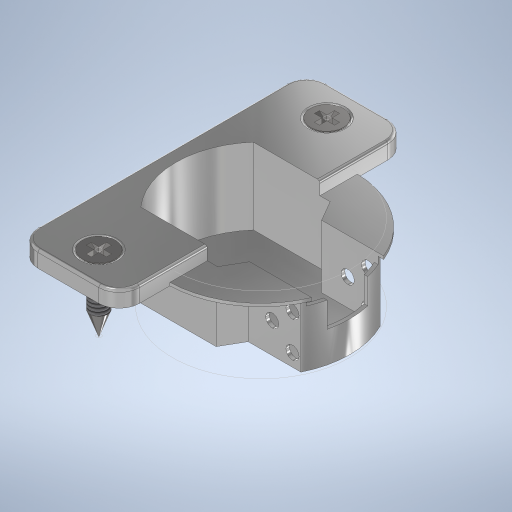
# Autodesk Inventor part: Cup for hinge with wood screws
Saved by Autodesk Inventor 2024 (Build 280153000, 153)
## iProperties
Created: 2007-06-13
Document SubType Name: Modeling
Designer: G.K.
Authority: Design by UAB Čeli APS
Material: Steel
Mass: 17.6743 g
Surface Area: 66.7103 cm^2
Volume: 2.2515 cm^3
Density: 7.85 g/cm^3
Appearance: Chrome - Polished
Part Number: Cup for hinge with wood screws
Perskaiciuoti: 1
Mase: 0.01767427
Autodesk Inventor part; units mm, degrees
ref_plane "YZ Plane" through (0, 0, 0) normal (1, 0, 0) x (0, 1, 0)
sketch "Sketch1" plane through (0, 0, 0) normal (0, 0, 1) x (1, 0, 0)
  line L0 (-10, -28.5) -> (10, -28.5)
  line L1 (10, -28.5) -> (10, 28.5)
  line L2 (10, 28.5) -> (-10, 28.5)
  line L3 (-10, 28.5) -> (-10, -28.5)
  point P0 (0, 0)
  point P1 (-10, 0)
  point P2 (0, 28.5)
  dimension "d0" = 20
  dimension "d1" = 57
  constraints: 8 end point, 2 midpoint, 2 parallel, 1 horizontal, 1 horizontal alignment, 1 perpendicular, 1 vertical alignment
  measures "d0" distance between parallel lines of L1 L3
  measures "d1" distance of L2.end L0.start
extrude "Extrusion1" add sketch "Sketch1" along normal blind 3.2
sketch "Sketch2" plane through (0, 0, 3.2) normal (0, 0, 1) x (1, 0, 0)
  line L0 (-10, -28.5) -> (-10, 28.5) projected
  line L1 (10, 28.5) -> (10, -28.5) projected
  line L2 (-10, 28.5) -> (10, 28.5) projected
  line L3 (0, 22.5) -> (0, -22.5) construction
  line L4 (-10, 0) -> (10, 0) construction
  point P0 (0, 0)
  dimension "d4" = 45
  constraints: 4 end point, 3 midpoint, 1 perpendicular, 1 symmetric about line
  measures "d4" distance of L3.start L3.end
hole "Hole1" at (0, -22.5, 3.2) at (0, 22.5, 3.2) direction (0, 0, -1) diameter 4.3 end through all countersink diameter 7 countersink angle 90
fillet "Fillet1" radius 0.5 4 edges at (0, 26, 3.2) (0, -19, 3.2) (0, -20.35, 1.85) (0, 24.65, 1.85)
fillet "Fillet1" radius 4 4 edges at (10, -28.5, 1.6) (-10, -28.5, 1.6) (-10, 28.5, 1.6) (10, 28.5, 1.6)
fillet "Fillet2" radius 0.5 8 edges at (-10, 0, 3.2) (-8.8284, 27.3284, 3.2) (0, 28.5, 3.2) (8.8284, 27.3284, 3.2) (10, 0, 3.2) (8.8284, -27.3284, 3.2) (0, -28.5, 3.2) (-8.8284, -27.3284, 3.2)
shell "Shell1" thickness 0.7 removed faces 1 at (6.9997, 6.8654, 0)
sketch "Sketch3" plane through (0, 0, 0) normal (0, 0, -1) x (-1, 0, 0)
  line L0 (-10, -24.5) -> (-10, 24.5) projected
  arc A0 (-10, 18.4932) -> (-10, -18.4932) centre (-9.5, 0) ccw
  line L1 (-39.6485, 0) -> (14.7113, 0)
  point P0 (0, 0)
  dimension "d16" = 18.5
  dimension "d17" = 0.5
  constraints: 3 point on line, 2 end point, 2 point on circle, 1 centre point, 1 horizontal, 2 other
  measures "d16" radius of A0
  measures "d17" distance from line of L0 A0.centre
extrude "Extrusion2" add sketch "Sketch3" against normal blind 0.6
sketch "Sketch4" plane through (0, 0, 0) normal (0, 0, -1) x (-1, 0, 0)
  line L0 (-14.7486, 7.8) -> (-25.1656, 7.8)
  arc A0 (-25.1656, 7.8) -> (-27, 0) centre (-9.5, 0) ccw
  arc A1 (-27, 0) -> (-25.1656, -7.8) centre (-9.5, 0) ccw
  line L1 (-25.1656, -7.8) -> (-14.7486, -7.8)
  line L2 (-12.4392, 11.8) -> (-14.7486, 7.8)
  line L3 (3.4232, 11.8) -> (-12.4392, 11.8)
  line L4 (-14.7486, -7.8) -> (-12.4392, -11.8)
  line L5 (-12.4392, -11.8) -> (3.4232, -11.8)
  arc A2 (3.4232, -11.8) -> (3.4232, 11.8) centre (-9.5, 0) ccw
  point P0 (0, 0)
  constraints: 12 end point, 6 point on circle, 4 horizontal, 3 centre point, 17 other
extrude "Extrusion3" add sketch "Sketch4" along normal blind 12.5
sketch "Sketch5" plane through (0, 0, 0) normal (0, 0, 1) x (1, 0, 0)
  line L0 (9.3, -11.8) -> (9.3, 11.8) projected
  line L1 (-3.4232, 11.8) -> (9.3, 11.8) projected
  arc A0 (-3.4232, 11.8) -> (-3.4232, -11.8) centre (9.5, 0) ccw projected
  line L2 (9.3, -11.8) -> (-3.4232, -11.8) projected
  point P0 (0, 0)
extrude "Extrusion4" add sketch "Sketch5" along normal up to surface (2.5 mm away)
sketch "Sketch6" plane through (0, 0, 3.2) normal (0, 0, 1) x (1, 0, 0)
  arc A0 (-3.4232, 11.8) -> (-3.4232, -11.8) centre (9.5, 0) ccw projected
  line L0 (9.3, 11.8) -> (-3.4232, 11.8) projected
  line L1 (12.4392, 11.8) -> (9.3, 11.8) projected
  line L2 (14.7486, 7.8) -> (12.4392, 11.8) projected
  line L3 (25.1656, 7.8) -> (14.7486, 7.8) projected
  line L4 (-3.4232, -11.8) -> (9.3, -11.8) projected
  line L5 (9.3, -11.8) -> (12.4392, -11.8) projected
  line L6 (12.4392, -11.8) -> (14.7486, -7.8) projected
  line L7 (14.7486, -7.8) -> (25.1656, -7.8) projected
  arc A1 (25.1656, -7.8) -> (25.1656, 7.8) centre (9.5, 0) ccw projected
  arc A2 (-3.1107, 11.1) -> (-3.1107, -11.1) centre (9.5, 0) ccw
  line L8 (-3.1107, -11.1) -> (9.3, -11.1)
  line L9 (9.3, -11.1) -> (12.035, -11.1)
  line L10 (12.035, -11.1) -> (14.3444, -7.1)
  line L11 (14.3444, -7.1) -> (24.726, -7.1)
  arc A3 (24.726, -7.1) -> (24.726, 7.1) centre (9.5, 0) ccw
  line L12 (24.726, 7.1) -> (14.3444, 7.1)
  line L13 (14.3444, 7.1) -> (12.035, 11.1)
  line L14 (12.035, 11.1) -> (9.3, 11.1)
  line L15 (9.3, 11.1) -> (-3.1107, 11.1)
  dimension "d24" = 0.7
  constraints: 16 end point, 4 point on circle, 2 centre point, 9 other
  measures "d24" radial gap between concentric circles of A2 A0
extrude "Extrusion5" cut sketch "Sketch6" against normal blind 15 contours L15 L14 L13 L12 A3 L11 L10 L9 L8 A2
sketch "Sketch7" plane through (0, 0, 0.6) normal (0, 0, 1) x (1, 0, 0)
  arc A0 (10, -18.4932) -> (10, 18.4932) centre (9.5, 0) ccw projected
  line L0 (14.3444, 7.1) -> (24.726, 7.1) projected
  line L1 (24.726, -7.1) -> (14.3444, -7.1) projected
  line L2 (24, 7.1) -> (28, 7.1)
  line L3 (28, 7.1) -> (28, -7.1)
  line L4 (28, -7.1) -> (24, -7.1)
  line L5 (24, -7.1) -> (24, 7.1)
  point P0 (0, 0)
  dimension "d27" = 4
  constraints: 8 end point, 2 parallel, 1 collinear, 1 horizontal, 1 perpendicular, 1 point on line, 1 tangent
  measures "d27" distance between parallel lines of L5 L3
extrude "Extrusion6" cut sketch "Sketch7" against normal blind 2
sketch "Sketch8" plane through (0, 0, -1.4) normal (0, 0, 1) x (1, 0, 0)
  arc A0 (25.495, -7.1) -> (25.495, 7.1) centre (9.5, 0) ccw projected
  line L0 (-17.4, 0) -> (34.4, 0) projected
  line L1 (23, 4) -> (27, 4)
  line L2 (27, 4) -> (27, -4)
  line L3 (27, -4) -> (23, -4)
  line L4 (23, -4) -> (23, 4)
  point P0 (0, 0)
  dimension "d30" = 8
  dimension "d31" = 4
  constraints: 8 end point, 2 parallel, 1 horizontal, 1 perpendicular, 1 tangent, 1 other
  measures "d30" distance between parallel lines of L3 L1
  measures "d31" distance between parallel lines of L2 L4
extrude "Extrusion7" cut sketch "Sketch8" against normal blind 5
sketch "Sketch9" plane through (14.7486, 7.8, -12.5) normal (0, 1, 0) x (1, 0, 0)
  line L0 (10.417, 0) -> (0, 0) projected
  line L1 (10.417, -12.5) -> (10.417, 0) projected
  line L2 (8.7514, -9.5) -> (8.7514, -2.5) construction
  line L3 (8.7514, -9.5) -> (4.7514, -6) construction
  line L4 (4.7514, -6) -> (8.7514, -2.5) construction
  line L5 (4.7514, -6) -> (8.7514, -6) construction
  line L6 (-24.7486, -12.5) -> (-24.7486, -15.2) projected
  point P0 (-14.7486, -12.5)
  dimension "d35" = 7
  dimension "d36" = 4
  dimension "d37" = 6
  dimension "d38" = 29.5
  constraints: 8 end point, 1 horizontal, 1 midpoint, 1 parallel
  measures "d35" distance of L2.start L2.end
  measures "d36" distance from line of L3.end L2
  measures "d37" distance from line of L3.end L0
  measures "d38" distance from line of L6 L3.end
hole "Hole2" at (23.5, 7.8, -10) at (19.5, 7.8, -6.5) at (23.5, 7.8, -3) direction (0, -1, 0) diameter 2.6 end through all
sketch "Sketch13" plane through (0, 0, 0) normal (0, 0, -1) x (-1, 0, 0)
  arc A0 (-25.495, -7.1) -> (-25.1656, -7.8) centre (-9.5, 0) ccw projected
  circle A1 centre (-9.5, 0) radius 17.5
  point P0 (0, 0)
  dimension "d76" = 35
  constraints: 1 centre point, 1 coincident
  measures "d76" diameter of A1
extrude "Extrusion9" add sketch "Sketch13" along normal blind 13 and the other way blind 2 separate body
ref_plane "Plane" through (32, 0, 0) normal (1, 0, 0) x (0, 1, 0)
ref_plane "Work Plane2" through (0, 22.5, -57.2917) normal (0, -1, 0) x (0, 0, 1)
sketch "Sketch10" plane through (0, 22.5, -57.2917) normal (0, -1, 0) x (0, 0, 1)
  line L0 (60.4917, -3.7071) -> (60.4917, 3.7071) projected
  line L1 (60.3917, -3.25) -> (58.8917, -1.75)
  line L2 (58.8917, -1.75) -> (50.2997, -1.75)
  line L3 (50.2997, -1.75) -> (45.4917, 0)
  line L4 (45.4917, 0) -> (60.4917, 0)
  line L5 (60.4917, 0) -> (60.4917, -3.25)
  line L6 (60.4917, -3.25) -> (60.3917, -3.25)
  point P0 (57.2917, 0)
  dimension "d56" = 3.5
  dimension "d57" = 15
  dimension "d58" = 0.1
  dimension "d59" = 6.5
  dimension "d60" = 20
  dimension "d61" = 45
  constraints: 12 end point, 2 perpendicular, 1 horizontal, 1 midpoint, 1 parallel
  measures "d56" diameter of L2 L4
  measures "d57" distance of L3.end L4.end
  measures "d58" distance of L5.end L1.start
  measures "d59" diameter of L6 L4
  measures "d60" angle of L4 L3
  measures "d61" angle of L4 L1
revolve "Wood screw Revolution1" add sketch "Sketch10" angle 360 about axis through (0, 22.5, -11.8) along (0, 0, 1) separate body
sketch "Sketch11" plane through (0, 22.5, -57.2917) normal (0, -1, 0) x (0, 0, 1)
  line L0 (60.4917, -2) -> (58.9917, -0.5)
  line L1 (58.9917, -0.5) -> (58.9917, 0.5)
  line L2 (58.9917, 0.5) -> (60.4917, 2)
  line L3 (60.4917, 2) -> (60.4917, -2)
  point P0 (57.2917, 0)
  point P1 (60.4917, 0)
  point P2 (60.4917, 0)
  dimension "d63" = 4
  dimension "d64" = 90
  dimension "d65" = 1.5
  constraints: 8 end point, 1 parallel, 1 vertical
  measures "d63" distance of L2.end L0.start
  measures "d64" angle of L2 L0
  measures "d65" distance between parallel lines of L3 L1
extrude "Wood screw Extrusion8" cut sketch "Sketch11" along normal mid plane 1 bodies 3
pattern_circular "Wood screw Circular Pattern1" count 2 over 90 about axis through (0, 22.5, -2.696) along (0, 0, -1) of "Wood screw Extrusion8" bodies 3
thread "Wood screw Thread1" size "M4x0.7" class "6g" standard "ANSI Metric M Profile" full length
sketch "Sketch12" plane through (0, 22.5, -57.2917) normal (0, -1, 0) x (0, 0, 1)
  line L0 (57.2917, 0) -> (45.7917, 0)
  line L1 (45.7917, 0) -> (45.7917, 0.5)
  line L2 (45.7917, 0.5) -> (57.2917, 0.5)
  line L3 (57.2917, 0.5) -> (57.2917, 0)
  line L4 (57.2917, 0.5) -> (60.5009, 0.5)
  line L5 (60.5009, 0.5) -> (60.5009, 0)
  line L6 (60.5009, 0) -> (57.2917, 0)
  dimension "d73" = 11.5
  dimension "d74" = 0.5
  constraints: 14 end point, 4 perpendicular, 2 parallel, 1 horizontal
  measures "d73" distance of L0.start L0.end
  measures "d74" distance of L0.end L1.end
revolve "Wood screw hole Revolution2" add sketch "Sketch12" angle 360 about axis through (0, 22.5, 0) along (0, 0, -1) separate body
mirror "Wood screw Mirror1" about plane through (0, 0, 0) normal (0, 1, 0) bodies 3
mirror "Wood screw hole Mirror2" about plane through (0, 0, 0) normal (0, 1, 0) bodies 4
sketch "Sketch14" plane through (0, 22.5, -57.2917) normal (0, -1, 0) x (0, 0, 1)
  line L0 (57.2917, -4.25) -> (48.2917, -4.25) construction
  line L1 (48.2917, -4.25) -> (48.2917, 0) construction
  line L2 (48.2917, 0) -> (57.2917, 0)
  line L3 (57.2917, 0) -> (57.2917, -4.25)
  line L4 (48.2917, 0) -> (48.2917, -3.85)
  line L5 (50.0917, -4.25) -> (50.0917, -3.85)
  line L6 (50.0917, -3.85) -> (51.8917, -4.25)
  line L7 (51.8917, -3.85) -> (53.6917, -4.25)
  line L8 (53.6917, -4.25) -> (53.6917, -3.85)
  line L9 (53.6917, -3.85) -> (55.4917, -4.25)
  line L10 (55.4917, -4.25) -> (55.4917, -3.85)
  line L11 (55.4917, -3.85) -> (57.2917, -4.25)
  line L12 (51.8917, -4.25) -> (51.8917, -3.85)
  line L13 (50.0917, -4.25) -> (48.2917, -3.85)
  point P0 (57.2917, 0)
  point P1 (57.2917, -4.5)
  dimension "d79" = 8.5
  dimension "d80" = 9
  dimension "d81" = 0.4
  dimension "d82" = 1.8
  constraints: 28 end point, 13 parallel, 5 point on line, 1 horizontal, 1 perpendicular
  measures "d79" diameter of L0 L2
  measures "d80" distance between parallel lines of L3 L1
  measures "d81" distance of L13.start L5.end
  measures "d82" distance between parallel lines of L1 L5
revolve "Knock-in Revolution3" [suppressed]
revolve "Knock-in hole Revolution4" [suppressed]
mirror "Knock-in Mirror3" [suppressed]
mirror "Knock-in hole Mirror4" [suppressed]
sketch "Sketch15" plane through (0, 22.5, -57.2917) normal (0, -1, 0) x (0, 0, 1)
  line L0 (57.2917, 0) -> (46.2917, 0)
  line L1 (46.2917, 0) -> (46.2917, 4)
  line L2 (46.2917, 4) -> (57.2917, 4)
  line L3 (57.2917, 4) -> (57.2917, 0)
  line L4 (57.2917, 0) -> (60.6191, 0)
  line L5 (60.6191, 0) -> (60.6191, 4)
  line L6 (60.6191, 4) -> (57.2917, 4)
  dimension "d84" = 11
  dimension "d85" = 4
  constraints: 14 end point, 3 parallel, 3 perpendicular, 1 horizontal
  measures "d84" distance of L0.start L0.end
  measures "d85" distance of L0.end L1.end
